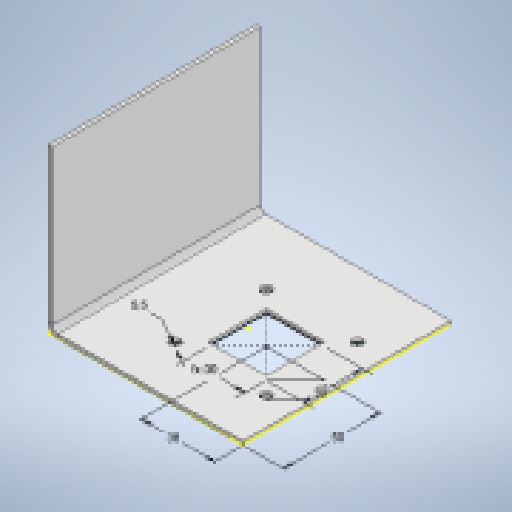
# Autodesk Inventor part: PNS 754 FDS 1200 FLANGE 2 down
Saved by Autodesk Inventor 2025 (Build 290162010, 162A)
## iProperties
Created: 2025-06-24
Part Number: PNS 754 FDS 1200 FLANGE 2 down
Material: Stainless Steel
Description: DIE16(5)|\ 90°|corrY -___°|X_____|bom___
Document SubType Name: Sheet Metal
Designer: pokla
Mass: 971.211 g
Surface Area: 1239.79 cm^2
Volume: 121.401 cm^3
Density: 8 g/cm^3
Flat Pattern Width: 18.0202 cm
Flat Pattern Length: 10.7 cm
Flat Pattern Area: 192.816 cm^2
Sheet Metal Rule: AISI304 2mm Die16
Sheet Metal Width: 180,202 mm
Sheet Metal Length: 107,000 mm
Sheet Metal Area: 19281,613 mm^2
Appearance: Default
d177: 30,000 mm
d178: 30,000 mm
d191: 30,000 mm
d192: 30,000 mm
Author: user
Autodesk Inventor part; units mm, degrees
ref_plane "YZ Plane" through (0, 0, 0) normal (1, 0, 0) x (0, 1, 0)
ref_plane "XZ Plane" through (0, 0, 0) normal (0, 1, 0) x (-1, 0, 0)
ref_plane "XY Plane" through (0, 0, 0) normal (0, 0, 1) x (1, 0, 0)
sketch "Sketch1" plane through (0, 0, 0) normal (0, 0, 1) x (1, 0, 0)
  line L0 (-50, -53.5) -> (50, -53.5)
  line L1 (50, -53.5) -> (50, 53.5)
  line L2 (50, 53.5) -> (-50, 53.5)
  line L3 (-50, 53.5) -> (-50, -53.5)
  line L4 (-50, -53.5) -> (50, 53.5) construction
  line L5 (50, -53.5) -> (-50, 53.5) construction
  point P0 (0, 0)
  dimension "d154" = 100
  dimension "d155" = 107
  measures "d154" distance of L1.end L2.end
  measures "d155" distance of L0.end L1.end
extrude "Plate5" add sketch "Sketch1" along normal blind 2
sketch "Sketch10" plane through (0, 0, 0) normal (0, 0, -1) x (-1, 0, 0)
  line L0 (3, -30.5) -> (-27, -30.5)
  line L1 (-27, -30.5) -> (-27, -0.5)
  line L2 (-27, -0.5) -> (3, -0.5)
  line L3 (3, -0.5) -> (3, -30.5)
  line L4 (3, -30.5) -> (-27, -0.5) construction
  line L5 (-27, -30.5) -> (3, -0.5) construction
  circle A0 centre (11.4853, -38.9853) radius 2.75
  circle A1 centre (-35.4853, -38.9853) radius 2.75
  circle A2 centre (-35.4853, 7.9853) radius 2.75
  circle A3 centre (11.4853, 7.9853) radius 2.75
  circle A4 centre (-12, -15.5) radius 33.2132 construction
  line L6 (-27, -30.5) -> (-35.4853, -38.9853) construction
  line L7 (-50, -53.5) -> (-50, 53.5) projected
  line L8 (50, -53.5) -> (-50, -53.5) projected
  line L9 (50, 53.5) -> (50, -53.5) projected
  line L10 (-50, 53.5) -> (50, 53.5) projected
  point P0 (0, 0)
  dimension "d187" = 30
  dimension "d188" = 30
  dimension "d189" = 5.5
  dimension "d190" = 12
  dimension "d196" = 38
  dimension "d198" = 69
  constraints: 14 end point, 5 centre point, 4 point on circle, 4 point on line, 3 equal radius, 2 midpoint, 2 parallel, 1 coincident, 1 horizontal, 1 perpendicular
  measures "d187" distance of L3.end L0.end
  measures "d188" distance of L0.end L2.start
  measures "d189" diameter of A0
  measures "d190" distance of L6.end L0.end
  measures "d196" distance from line of L7 point (-12, -15.5)
  measures "d198" distance from line of L10 point (-12, -15.5)
extrude "Cut2" cut sketch "Sketch10" against normal through all contours L0 L1 L2 L3 | A0 | A1 | A2 | A3
sketch "Sketch7" plane through (-48, -53.5, 0) normal (-1, 0, 0) x (0, -1, 0)
  line L0 (-107, 0) -> (0, 0)
  line L1 (0, 0) -> (0, 84)
  line L2 (0, 84) -> (-107, 84)
  line L3 (-107, 84) -> (-107, 0)
  constraints: 6 end point, 1 horizontal, 1 perpendicular, 1 vertical
edge flange "Flange3" height 84 angle 90 thickness 2 bend radius 2.75 thickness toward (-1, 0, 0) relief round relief width 2 relief depth 1 edges at (-50, 0, 2) wall of the first edge with corners at (-48, 53.5, 0) (-48, -53.5, 0) (-48, -53.5, 84) (-48, 53.5, 84)
bend "Bend3"
corner "Corner3"
body "Solid3"
